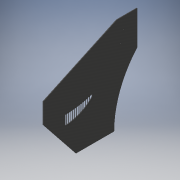
# Autodesk Inventor part: end_plate
Saved by Autodesk Inventor 2018 (Build 220112000, 112)
## iProperties
Created: 2017-10-22
Part Number: end_plate
Material: CFRP
Document SubType Name: Modeling
Designer: ku_sk
Density: 1.43 g/cm^3
Appearance: カーボンファイバー
Author: ku_sk
Autodesk Inventor part; units mm, degrees
ref_plane "YZ Plane" through (0, 0, 0) normal (1, 0, 0) x (0, 1, 0)
ref_plane "XY Plane" through (0, 0, 0) normal (0, 0, 1) x (1, 0, 0)
sketch "スケッチ1" plane through (0, 0, 0) normal (1, 0, 0) x (0, 1, 0)
  line L0 (-700, 170) -> (-700, 450)
  line L1 (-700, 450) -> (-400, 690)
  line L2 (-400, 690) -> (-250, 690)
  line L3 (-250, 690) -> (0, 150)
  line L4 (0, 150) -> (0, 0)
  line L5 (0, 0) -> (-250, 0)
  arc A0 (-250, 0) -> (-700, 170) centre (-700, -510.5882) ccw
  dimension "d0" = 690
  dimension "d1" = 280
  dimension "d2" = 240
  dimension "d3" = 300
  dimension "d4" = 150
  dimension "d5" = 700
  dimension "d6" = 250
  dimension "d7" = 150
  constraints: 12 end point, 2 perpendicular, 2 point on circle, 1 centre point, 1 coincident, 1 horizontal, 1 line through centre, 1 parallel
  measures "d0" distance between parallel lines of L5 L2
  measures "d1" distance of L0.start L0.end
  measures "d2" distance from line of L0.end L2
  measures "d3" distance from line of L1.end L0
  measures "d4" distance of L3.end L4.end
  measures "d5" distance between parallel lines of L0 L4
  measures "d6" distance of L4.end L5.end
  measures "d7" distance of L1.end L2.end
extrude "押し出し1" add sketch "スケッチ1" along normal blind 5
sketch "スケッチ2" plane through (5, 0, 0) normal (1, 0, 0) x (0, 0, -1)
  circle A0 centre (-100, -87) radius 2.5
  line L0 (0, 0) -> (-150, 0) projected
  line L1 (0, -250) -> (0, 0) projected
  circle A1 centre (-125, -164) radius 2.5
  dimension "d10" = 87
  dimension "d11" = 100
  dimension "d12" = 5
  dimension "d13" = 164
  dimension "d14" = 125
  dimension "d15" = 5
  constraints: 2 centre point
  measures "d10" distance from line of L0 A0.centre
  measures "d11" distance from line of L1 A0.centre
  measures "d12" diameter of A0
  measures "d13" distance from line of L0 A1.centre
  measures "d14" distance from line of L1 A1.centre
  measures "d15" diameter of A1
extrude "押し出し2" cut sketch "スケッチ2" against normal through all
sketch "スケッチ4" plane through (5, 0, 0) normal (1, 0, 0) x (0, 0, -1)
  arc A0 (-530, -415) -> (-330, -380) centre (-530, 173.9286) ccw
  line L0 (-530, -415) -> (-530, -485)
  line L1 (-690, -250) -> (-690, -400) projected
  arc A1 (-530, -485) -> (-330, -400) centre (-530, -207.2059) ccw
  line L2 (-330, -380) -> (-330, -400)
  point P0 (0, 0)
  dimension "d18" = 70
  dimension "d19" = 160
  dimension "d20" = 20
  dimension "d21" = 15
  dimension "d22" = 200
  dimension "d23" = 35
  constraints: 4 end point, 4 point on circle, 2 centre point, 2 line through centre, 1 parallel, 1 vertical
  measures "d18" distance of L0.start L0.end
  measures "d19" distance between parallel lines of L1 L0
  measures "d20" distance of L2.start L2.end
  measures "d21" vertical distance of L1.end L0.start
  measures "d22" distance between parallel lines of L0 L2
  measures "d23" vertical distance of L0.start L2.start
extrude "押し出し3" cut sketch "スケッチ4" against normal through all
ref_plane "作業平面1" through (0, -500, 0) normal (0, 1, 0) x (-1, 0, 0)
sketch "スケッチ5" plane through (0, -500, 0) normal (0, 1, 0) x (-1, 0, 0)
  line L0 (0, 512.8397) -> (-0.866, 512.3397)
  line L1 (-0.866, 512.3397) -> (-5, 519.5)
  line L2 (-5, 519.5) -> (-4.134, 520)
  line L3 (-4.134, 520) -> (0, 512.8397)
  line L4 (0, 530) -> (0, 330) projected
  line L5 (-4.134, 506) -> (0, 498.8397)
  line L6 (0, 498.8397) -> (-0.866, 498.3397)
  line L7 (-0.866, 498.3397) -> (-5, 505.5)
  line L8 (-5, 505.5) -> (-4.134, 506)
  line L9 (-4.134, 492) -> (0, 484.8397)
  line L10 (0, 484.8397) -> (-0.866, 484.3397)
  line L11 (-0.866, 484.3397) -> (-5, 491.5)
  line L12 (-5, 491.5) -> (-4.134, 492)
  line L13 (-4.134, 478) -> (0, 470.8397)
  line L14 (0, 470.8397) -> (-0.866, 470.3397)
  line L15 (-0.866, 470.3397) -> (-5, 477.5)
  line L16 (-5, 477.5) -> (-4.134, 478)
  line L17 (-4.134, 464) -> (0, 456.8397)
  line L18 (0, 456.8397) -> (-0.866, 456.3397)
  line L19 (-0.866, 456.3397) -> (-5, 463.5)
  line L20 (-5, 463.5) -> (-4.134, 464)
  line L21 (-4.134, 450) -> (0, 442.8397)
  line L22 (0, 442.8397) -> (-0.866, 442.3397)
  line L23 (-0.866, 442.3397) -> (-5, 449.5)
  line L24 (-5, 449.5) -> (-4.134, 450)
  line L25 (-4.134, 436) -> (0, 428.8397)
  line L26 (0, 428.8397) -> (-0.866, 428.3397)
  line L27 (-0.866, 428.3397) -> (-5, 435.5)
  line L28 (-5, 435.5) -> (-4.134, 436)
  line L29 (-4.134, 422) -> (0, 414.8397)
  line L30 (0, 414.8397) -> (-0.866, 414.3397)
  line L31 (-0.866, 414.3397) -> (-5, 421.5)
  line L32 (-5, 421.5) -> (-4.134, 422)
  line L33 (-4.134, 408) -> (0, 400.8397)
  line L34 (0, 400.8397) -> (-0.866, 400.3397)
  line L35 (-0.866, 400.3397) -> (-5, 407.5)
  line L36 (-5, 407.5) -> (-4.134, 408)
  line L37 (-4.134, 394) -> (0, 386.8397)
  line L38 (0, 386.8397) -> (-0.866, 386.3397)
  line L39 (-0.866, 386.3397) -> (-5, 393.5)
  line L40 (-5, 393.5) -> (-4.134, 394)
  line L41 (-4.134, 380) -> (0, 372.8397)
  line L42 (0, 372.8397) -> (-0.866, 372.3397)
  line L43 (-0.866, 372.3397) -> (-5, 379.5)
  line L44 (-5, 379.5) -> (-4.134, 380)
  line L45 (-4.134, 366) -> (0, 358.8397)
  line L46 (0, 358.8397) -> (-0.866, 358.3397)
  line L47 (-0.866, 358.3397) -> (-5, 365.5)
  line L48 (-5, 365.5) -> (-4.134, 366)
  line L49 (-4.134, 352) -> (0, 344.8397)
  line L50 (0, 344.8397) -> (-0.866, 344.3397)
  line L51 (-0.866, 344.3397) -> (-5, 351.5)
  line L52 (-5, 351.5) -> (-4.134, 352)
  line L53 (-5, 150) -> (-5, 690) projected
  point P0 (0, 0)
  point P1 (-5, 530)
  point P2 (-5, 399.75)
  point P3 (-5, 389.75)
  dimension "d30" = 1
  dimension "d34" = 14
  dimension "d42" = 30
  dimension "d43" = 10
  constraints: 104 end point, 3 perpendicular, 1 point on line, 1 vertical, 98 other
  measures "d30" distance of L0.start L0.end
  measures "d34" distance of L2.end L5.start
  measures "d42" angle to the sketch y axis of L1
  measures "d43" vertical distance of point (-5, 530) L2.end
extrude "押し出し5" add sketch "スケッチ5" along normal blind 130 contours L0 L1 L2 L3 | L6 L7 L8 L5 | L10 L11 L12 L9 | L14 L15 L16 L13 | L18 L19 L20 L17 | L22 L23 L24 L21 | L26 L27 L28 L25 | L30 L31 L32 L29 | L34 L35 L36 L33 | L38 L39 L40 L37 | L42 L43 L44 L41 | L46 L47 L48 L45 | L50 L51 L52 L49
